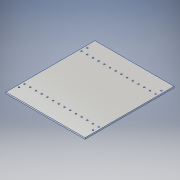
# Autodesk Inventor part: CustomBasePlate
Saved by Autodesk Inventor 2016 (Build 200138000, 138)
## iProperties
Created: 2015-08-31
Part Number: CustomBasePlate
Material: Aluminum 6061
Document SubType Name: Modeling
Designer: Tim
Density: 2.7 g/cm^3
Appearance: Aluminum - Flat
Author: Tim
Autodesk Inventor part; units mm, degrees
ref_plane "YZ Plane" through (0, 0, 0) normal (1, 0, 0) x (0, 1, 0)
ref_plane "XZ Plane" through (0, 0, 0) normal (0, 1, 0) x (-1, 0, 0)
ref_plane "XY Plane" through (0, 0, 0) normal (0, 0, 1) x (1, 0, 0)
sketch "Sketch1" plane through (0, 0, 0) normal (0, 1, 0) x (-1, 0, 0)
  line L0 (90.125, -125.756) -> (-131.875, -125.756)
  line L1 (-131.875, -125.756) -> (-131.875, 104.244)
  line L2 (-131.875, 104.244) -> (90.125, 104.244)
  line L3 (90.125, 104.244) -> (90.125, -125.756)
  line L4 (83.125, 94.744) -> (-124.875, -97.256) construction
  line L5 (-124.875, 94.744) -> (83.125, -97.256) construction
  circle A0 centre (83.125, -97.256) radius 2
  circle A1 centre (-124.875, -97.256) radius 2
  circle A2 centre (-124.875, 94.744) radius 2
  circle A3 centre (83.125, 94.744) radius 2
  point P0 (0, 0)
  point P1 (-20.875, -125.756)
  point P2 (90.125, -10.756)
  point P3 (-20.8729, -81.6668)
  point P4 (-124.8729, -81.6668)
  point P5 (-20.875, -1.256)
  dimension "d0" = 230
  dimension "d1" = 222
  dimension "d5" = 208
  dimension "d6" = 192
  dimension "d7" = 4
  dimension "d8" = 4
  dimension "d9" = 4
  dimension "d10" = 4
  constraints: 12 end point, 4 centre point, 4 coincident, 4 midpoint, 2 parallel, 1 horizontal, 1 perpendicular
  measures "d0" distance of L0.end L1.end
  measures "d1" distance of L1.end L2.end
  measures "d5" distance of L5.end L4.end
  measures "d6" distance of L5.end L4.start
  measures "d7" diameter of A0
  measures "d8" diameter of A1
  measures "d9" diameter of A2
  measures "d10" diameter of A3
extrude "Extrusion1" add sketch "Sketch1" along normal blind 4
sketch "Sketch2" plane through (0, 0, 0) normal (0, -1, 0) x (1, 0, 0)
  circle A0 centre (124.7852, -81.3481) radius 1.85 projected
  circle A1 centre (108.7852, -81.3481) radius 1.85 projected
  circle A2 centre (92.7863, -81.156) radius 1.85 projected
  circle A3 centre (76.7863, -81.156) radius 1.85 projected
  circle A4 centre (60.7863, -81.156) radius 1.85 projected
  circle A5 centre (44.7863, -81.156) radius 1.85 projected
  circle A6 centre (28.7863, -81.156) radius 1.85 projected
  circle A7 centre (12.7863, -81.156) radius 1.85 projected
  circle A8 centre (-3.2137, -81.156) radius 1.85 projected
  circle A9 centre (-19.2137, -81.156) radius 1.85 projected
  circle A10 centre (-35.2137, -81.156) radius 1.85 projected
  circle A11 centre (-51.2137, -81.156) radius 1.85 projected
  circle A12 centre (-67.2137, -81.156) radius 1.85 projected
  circle A13 centre (-83.2137, -81.156) radius 1.85 projected
  circle A14 centre (124.7852, 78.6519) radius 1.85 projected
  circle A15 centre (108.7852, 78.6519) radius 1.85 projected
  circle A16 centre (92.7852, 78.6519) radius 1.85 projected
  circle A17 centre (76.7852, 78.6519) radius 1.85 projected
  circle A18 centre (60.7852, 78.6519) radius 1.85 projected
  circle A19 centre (44.7852, 78.6519) radius 1.85 projected
  circle A20 centre (28.7852, 78.6519) radius 1.85 projected
  circle A21 centre (12.7852, 78.6519) radius 1.85 projected
  circle A22 centre (-3.2148, 78.6519) radius 1.85 projected
  circle A23 centre (-19.2148, 78.6519) radius 1.85 projected
  circle A24 centre (-35.2148, 78.6519) radius 1.85 projected
  circle A25 centre (-51.2148, 78.6519) radius 1.85 projected
  circle A26 centre (-67.2137, 78.844) radius 1.85 projected
  circle A27 centre (-83.2137, 78.844) radius 1.85 projected
  line L0 (228.7863, -90.756) -> (-187.2137, -90.756) projected
  line L1 (228.7863, -90.756) -> (-187.2137, -90.756) projected
  line L2 (-90.125, -125.756) -> (131.875, -125.756) projected
  line L3 (-187.2148, 88.2519) -> (228.7852, 88.2519) projected
  line L4 (131.875, 104.244) -> (-90.125, 104.244) projected
  point P0 (0, 0)
  dimension "d13" = 35
  dimension "d14" = 15.9922
  measures "d13" distance between parallel lines of L1 L2
  measures "d14" distance between parallel lines of L4 L3
hole "Hole1" at (124.7852, 0, 78.6519) at (108.7852, 0, 78.6519) at (92.7852, 0, 78.6519) at (76.7852, 0, 78.6519) at (60.7852, 0, 78.6519) at (44.7852, 0, 78.6519) at (28.7852, 0, 78.6519) at (12.7852, 0, 78.6519) at (-3.2148, 0, 78.6519) at (-19.2148, 0, 78.6519) at (-35.2148, 0, 78.6519) at (-51.2148, 0, 78.6519) at (-67.2137, 0, 78.844) at (-83.2137, 0, 78.844) at (-83.2137, 0, -81.156) at (-67.2137, 0, -81.156) at (-51.2137, 0, -81.156) at (-35.2137, 0, -81.156) at (-19.2137, 0, -81.156) at (-3.2137, 0, -81.156) at (12.7863, 0, -81.156) at (28.7863, 0, -81.156) at (44.7863, 0, -81.156) at (60.7863, 0, -81.156) at (76.7863, 0, -81.156) at (92.7863, 0, -81.156) at (108.7852, 0, -81.3481) at (124.7852, 0, -81.3481) direction (0, 1, 0) diameter 3.8 end through all
sketch "Sketch4" plane through (-90.125, 0, 104.244) normal (0, 0, 1) x (1, 0, 0)
  line L0 (222, 0) -> (0, 0) projected
  line L1 (222, 0) -> (0, 0) projected
  line L2 (222, 0) -> (222, 4) projected
  line L3 (0, 4) -> (222, 4) projected
  line L4 (0, 0) -> (0, 4) projected
  point P0 (90.125, 0)
extrude "Extrusion2" add sketch "Sketch4" along normal blind 20
body "Solid1"
